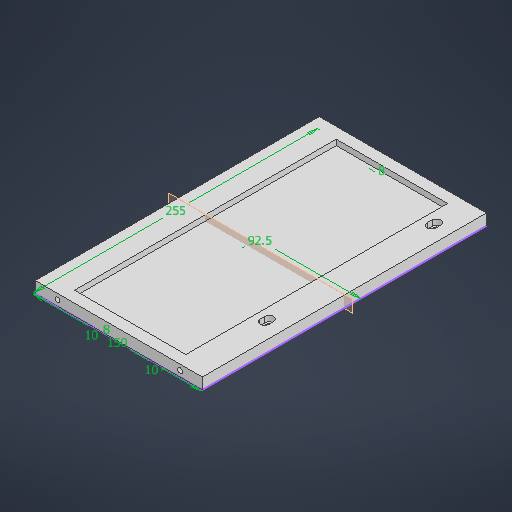
# Autodesk Inventor part: bottomplate
Saved by Autodesk Inventor 2025.1 (Build 291241000, 241)
## iProperties
Created: 2025-03-19
Part Number: bottomplate
Material: Generic
Document SubType Name: Modeling
Designer: m_kni
Density: 1 g/cm^3
Appearance: Default
Author: m_kni
Autodesk Inventor part; units mm, degrees
ref_plane "YZ Plane" through (0, 0, 0) normal (1, 0, 0) x (0, 1, 0)
ref_plane "XZ Plane" through (0, 0, 0) normal (0, 1, 0) x (-1, 0, 0)
ref_plane "XY Plane" through (0, 0, 0) normal (0, 0, 1) x (1, 0, 0)
sketch "Sketch1" plane through (0, 0, 0) normal (0, 1, 0) x (-1, 0, 0)
  line L0 (-74.8419, -127.4209) -> (75.1581, -127.4209)
  line L1 (75.1581, -127.4209) -> (75.1581, 127.5791)
  line L2 (75.1581, 127.5791) -> (-74.8419, 127.5791)
  line L3 (-74.8419, 127.5791) -> (-74.8419, -127.4209)
  line L4 (-74.8419, -127.4209) -> (75.1581, 127.5791) construction
  line L5 (75.1581, -127.4209) -> (-74.8419, 127.5791) construction
  line L6 (-74.8419, 0.0791) -> (-36.3419, 0.0791)
  line L7 (-41.3419, -127.4209) -> (-31.3419, -127.4209)
  line L8 (-31.3419, -127.4209) -> (-31.3419, 127.5791)
  line L9 (-31.3419, 127.5791) -> (-41.3419, 127.5791)
  line L10 (-41.3419, 127.5791) -> (-41.3419, -127.4209)
  line L11 (-41.3419, -127.4209) -> (-31.3419, 127.5791) construction
  line L12 (-31.3419, -127.4209) -> (-41.3419, 127.5791) construction
  line L13 (12.6581, -127.4209) -> (22.6581, -127.4209)
  line L14 (22.6581, -127.4209) -> (22.6581, 127.5791)
  line L15 (22.6581, 127.5791) -> (12.6581, 127.5791)
  line L16 (12.6581, 127.5791) -> (12.6581, -127.4209)
  line L17 (12.6581, -127.4209) -> (22.6581, 127.5791) construction
  line L18 (22.6581, -127.4209) -> (12.6581, 127.5791) construction
  line L19 (75.1581, 127.5791) -> (22.3444, 127.5791)
  line L20 (22.3444, 127.5791) -> (22.3444, 119.5791)
  line L21 (22.3444, 119.5791) -> (75.1581, 119.5791)
  line L22 (75.1581, 119.5791) -> (75.1581, 127.5791)
  line L23 (75.1581, -127.4209) -> (22.3444, -127.4209)
  line L24 (22.3444, -127.4209) -> (22.3444, -119.4209)
  line L25 (22.3444, -119.4209) -> (75.1581, -119.4209)
  line L26 (75.1581, -119.4209) -> (75.1581, -127.4209)
  line L27 (12.9719, -119.4209) -> (-31.3419, -119.4209)
  line L28 (-31.3419, -119.4209) -> (-31.3419, -127.4209)
  line L29 (-31.3419, -127.4209) -> (12.9719, -127.4209)
  line L30 (12.9719, -127.4209) -> (12.9719, -119.4209)
  line L31 (22.3444, 119.5791) -> (-31.3419, 119.5791)
  line L32 (-31.3419, 119.5791) -> (-31.3419, 127.5791)
  line L33 (-31.3419, 127.5791) -> (22.3444, 127.5791)
  line L34 (22.3444, 127.5791) -> (22.3444, 119.5791)
  point P0 (0, 0)
  point P1 (0.1581, 0.0791)
  point P2 (17.6581, 0.0791)
  point P3 (22.6581, -119.4209)
  point P4 (22.6581, 119.5791)
  point P5 (-31.3419, -119.4209)
  point P6 (12.6581, 119.5791)
  point P7 (12.6581, -119.4209)
  point P8 (-36.3419, -127.4209)
  dimension "d0" = 150
  dimension "d1" = 255
  dimension "d2" = 10
  dimension "d3" = 92.5
  dimension "d4" = 10
  dimension "d5" = 8
  dimension "d6" = 8
  constraints: 70 end point, 14 parallel, 8 horizontal, 8 midpoint, 7 perpendicular, 5 point on line
  measures "d0" distance of L2.end L1.end
  measures "d1" distance of L1.end L0.end
  measures "d2" distance of L9.end L8.end
  measures "d3" distance from line of point (17.658, 0.079) L3
  measures "d4" distance of L15.end L14.end
  measures "d5" distance of L20.end L19.end
  measures "d6" distance of L23.end L24.end
extrude "Extrusion1" add sketch "Sketch1" along normal blind 10
sketch "Sketch2" plane through (-75.1581, 0, 127.5791) normal (0, 0, 1) x (1, 0, 0)
  line L0 (0, 0) -> (0, 10) projected
  line L1 (150, 0) -> (150, 10) projected
  circle A0 centre (20, 5) radius 2.25
  circle A1 centre (130, 5) radius 2.25
  point P0 (75.1581, 0)
  point P1 (0, 5)
  point P2 (0, 5)
  point P3 (150, 5)
  dimension "d9" = 20
  dimension "d10" = 20
  dimension "d11" = 4.5
  dimension "d12" = 4.5
  constraints: 3 midpoint, 2 centre point, 2 coincident
  measures "d9" distance of point (20, 5) point (0, 5)
  measures "d10" horizontal distance of L1.start point (130, 5)
  measures "d11" diameter of A0
  measures "d12" diameter of A1
extrude "Extrusion2" cut sketch "Sketch2" against normal blind 10
ref_plane "Work Plane1" through (-75.1581, 0, 0.0791) normal (0, 0, 1) x (1, 0, 0)
mirror "Mirror1" about plane through (-75.1581, 0, 0.0791) normal (0, 0, 1) of "Extrusion2"
sketch "Sketch3" plane through (0, 0, 0) normal (0, -1, 0) x (1, 0, 0)
  line L0 (74.8419, -127.4209) -> (-75.1581, -127.4209) projected
  line L1 (74.8419, 127.5791) -> (74.8419, -127.4209) projected
  circle A0 centre (59.8419, 54.5791) radius 2.25
  circle A1 centre (59.8419, -95.4209) radius 2.25
  circle A2 centre (59.8419, -97.6709) radius 2.25
  circle A3 centre (59.8419, -93.1709) radius 2.25
  line L2 (62.0919, -93.1709) -> (62.0919, -97.6709)
  line L3 (57.5919, -93.1709) -> (57.5919, -97.6709)
  circle A4 centre (59.8419, 52.3291) radius 2.25
  circle A5 centre (59.8419, 56.8291) radius 2.25
  line L4 (57.5919, 56.8291) -> (57.5919, 52.3291)
  line L5 (62.0919, 56.8291) -> (62.0919, 52.3291)
  point P0 (0, 0)
  dimension "d15" = 32
  dimension "d16" = 15
  dimension "d17" = 150
  dimension "d19" = 4.5
  dimension "d20" = 4.5
  dimension "d21" = 4.5
  dimension "d22" = 4.5
  dimension "d23" = 4.5
  dimension "d24" = 4.5
  constraints: 12 point on circle, 8 end point, 6 centre point, 4 tangent, 1 coincident, 1 vertical
  measures "d15" distance from line of L0 point (59.842, -95.421)
  measures "d16" distance from line of L1 point (59.842, -95.421)
  measures "d17" distance of point (59.842, 54.579) point (59.842, -95.421)
  measures "d19" diameter of A0
  measures "d20" diameter of A1
  measures "d21" diameter of A2
  measures "d22" diameter of A3
  measures "d23" diameter of A4
  measures "d24" diameter of A5
extrude "Extrusion3" cut sketch "Sketch3" against normal blind 10
sketch "Sketch4" plane through (0, 10, 0) normal (0, 1, 0) x (1, 0, 0)
  line L0 (62.0919, 97.6709) -> (62.0919, 93.1709) projected
  arc A0 (57.5919, 93.1709) -> (62.0919, 93.1709) centre (59.8419, 93.1709) ccw projected
  line L1 (57.5919, 93.1709) -> (57.5919, 97.6709) projected
  arc A1 (62.0919, 97.6709) -> (57.5919, 97.6709) centre (59.8419, 97.6709) ccw projected
  line L2 (57.5919, -56.8291) -> (57.5919, -52.3291) projected
  arc A2 (62.0919, -52.3291) -> (57.5919, -52.3291) centre (59.8419, -52.3291) ccw projected
  line L3 (62.0919, -52.3291) -> (62.0919, -56.8291) projected
  arc A3 (57.5919, -56.8291) -> (62.0919, -56.8291) centre (59.8419, -56.8291) ccw projected
  line L4 (-75.1581, 127.4209) -> (-75.1581, -127.5791) projected
  line L5 (-75.1581, -127.5791) -> (74.8419, -127.5791) projected
  line L6 (74.8419, -127.5791) -> (74.8419, 127.4209) projected
  line L7 (74.8419, 127.4209) -> (-75.1581, 127.4209) projected
  circle A4 centre (59.8419, -56.8291) radius 4
  circle A5 centre (59.8419, -52.3291) radius 4
  line L8 (63.8419, -56.8291) -> (63.8419, -52.3291)
  line L9 (55.8419, -56.8291) -> (55.8419, -52.3291)
  circle A6 centre (59.8419, 93.1709) radius 4
  circle A7 centre (59.8419, 97.6709) radius 4
  line L10 (63.8419, 97.6709) -> (63.8419, 93.1709)
  line L11 (55.8419, 93.1709) -> (55.8419, 97.6709)
  point P0 (0, 0)
  point P1 (57.5919, 96.4781)
  point P2 (62.0919, 96.4781)
  dimension "d27" = 8
  dimension "d28" = 8
  dimension "d29" = 8
  dimension "d30" = 8
  constraints: 8 end point, 8 point on circle, 4 centre point, 4 coincident, 3 tangent, 2 vertical, 1 parallel
  measures "d27" diameter of A4
  measures "d28" diameter of A5
  measures "d29" diameter of A6
  measures "d30" diameter of A7
extrude "Extrusion4" cut sketch "Sketch4" against normal blind 5 contours A1 L1 A6 A7 L0 | A6 A7 L0 | L0 A7 L1 A6 | A7 A6 L1 A0 L0 | L0 A0 L1 A7 | A7 L10 A6 | L1 A7 A6 | A6 L11 A7 | A3 L3 A5 A4 L2 | A5 A4 L2 | A4 A5 L3 A2 L2 | A4 L9 A5 | L3 A4 A5 | A5 L8 A4
sketch "Sketch5" plane through (0, 10, 0) normal (0, 1, 0) x (1, 0, 0)
  line L0 (50, 117.5) -> (-50, 117.5)
  line L1 (-50, 117.5) -> (-50, -117.5)
  line L2 (-50, -117.5) -> (50, -117.5)
  line L3 (50, -117.5) -> (50, 117.5)
  line L4 (50, 117.5) -> (-50, -117.5) construction
  line L5 (-50, 117.5) -> (50, -117.5) construction
  point P0 (0, 0)
  dimension "d33" = 100
  dimension "d34" = 235
  constraints: 12 end point, 2 midpoint, 2 parallel, 1 horizontal, 1 perpendicular
  measures "d33" distance of L2.end L1.end
  measures "d34" distance of L1.end L0.end
extrude "Extrusion5" cut sketch "Sketch5" against normal up to surface (5 mm away)
body "Solid1"
